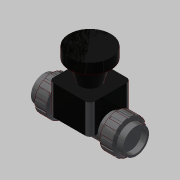
# Autodesk Inventor part: DIAPHRAGM VALVE MANUAL GLUED DN50
Saved by Autodesk Inventor 2017 (Build 210142000, 142)
## iProperties
Created: 2016-04-26
Part Number: DIAPHRAGM VALVE MANUAL GLUED DN50
Description: DKUIV
Document SubType Name: Modeling
Manufacturer: SEKISUI
Mass: 197.859 g
Surface Area: 285.44 cm^2
Volume: 153.379 cm^3
Density: 1.29 g/cm^3
Material: PVC
Appearance: Smooth - White(2)
Catalog Web Link: http://www.pocketbrewery.com
Title: BALL VALVE PVC-U TRD DN15
Autodesk Inventor part; units mm, degrees
ref_plane "YZ Plane" through (0, 0, 0) normal (1, 0, 0) x (0, 1, 0)
ref_plane "XZ Plane" through (0, 0, 0) normal (0, 1, 0) x (-1, 0, 0)
ref_plane "XY Plane" through (0, 0, 0) normal (0, 0, 1) x (1, 0, 0)
sketch "Sketch_1" plane through (0, 0, 0) normal (1, 0, 0) x (0, 1, 0)
  line L0 (116.9615, 0) -> (116.9615, -32.6667)
  line L1 (116.9615, -32.6667) -> (111.0167, -49)
  line L2 (111.0167, -49) -> (77.6193, -49)
  line L3 (77.6193, -49) -> (74.7393, -41.0872)
  line L4 (74.7393, -41.0872) -> (74.7393, -32.6667)
  line L5 (-74.7393, -32.6667) -> (-74.7393, -41.0872)
  line L6 (-74.7393, -41.0872) -> (-77.6193, -49)
  line L7 (-77.6193, -49) -> (-111.0167, -49)
  line L8 (-111.0167, -49) -> (-116.9615, -32.6667)
  line L9 (-116.9615, -32.6667) -> (-116.9615, 0)
  line L10 (-116.9615, 0) -> (116.9615, 0)
  line L11 (-77.6193, -49) -> (0, -49) construction
  line L12 (0, -49) -> (0, -50.7038) construction
  line L13 (-111.7446, -49) -> (-79.6193, -49)
  line L14 (-79.6193, -49) -> (-79.6193, -47)
  line L15 (-79.6193, -47) -> (-111.7446, -47)
  line L16 (-111.7446, -47) -> (-111.7446, -49)
  line L17 (79.6193, -49) -> (111.7446, -49)
  line L18 (111.7446, -49) -> (111.7446, -47)
  line L19 (111.7446, -47) -> (79.6193, -47)
  line L20 (79.6193, -47) -> (79.6193, -49)
  line L21 (-74.7393, -32.6667) -> (74.7393, -32.6667)
  point P0 (0, 0)
  point P1 (0, 0)
  point P2 (-94.318, -49)
  point P3 (95.682, -49)
  point P4 (0, 0)
  dimension "dimE" = 98
  dimension "d22" = 49
  dimension "d23" = 16.3333
  dimension "d24" = 20
  dimension "d27" = 42.2222
  dimension "d28" = 42.2222
  dimension "d52" = 20
  dimension "d53" = 2
  dimension "d54" = 2
  dimension "d55" = 2
  dimension "dimZ" = 190
  constraints: 44 end point, 6 parallel, 5 equal length, 5 horizontal, 5 perpendicular, 4 point on line, 3 collinear, 3 midpoint, 2 coincident
  measures "dimE" diameter of L2 L10
  measures "d22" distance from line of L0.start L2
  measures "d23" vertical distance of L0.end L1.end
  measures "d24" angle of L0 L1
  measures "d27" distance between parallel lines of L9 L5
  measures "d28" distance between parallel lines of L0 L4
  measures "d52" angle of L5 L6
  measures "d53" distance of L15.end L13.start
  measures "d54" distance from line of L6.end L14
  measures "d55" distance from line of L2.end L20
  measures "dimZ" distance of point (95.682, -49) point (-94.318, -49)
revolve "Revolution1" add sketch "Sketch_1" angle 360 about axis through (0, -116.9615, 0) along (0, 1, 0) contours L0 L1 L19 L20 L2 L3 L4 L21 L5 L6 L7 L14 L15 L8 L9 L10 | L1 L2 L20 L19 | L15 L14 L7 L8 | L8 L13 L16
sketch "Sketch11" plane through (0, 0, 0) normal (0, 0, 1) x (1, 0, 0)
  line L0 (-59.7393, 59.7393) -> (59.7393, 59.7393)
  line L1 (59.7393, 59.7393) -> (59.7393, -59.7393)
  line L2 (59.7393, -59.7393) -> (-59.7393, -59.7393)
  line L3 (-59.7393, -59.7393) -> (-59.7393, 59.7393)
  line L4 (59.7393, -59.7393) -> (-59.7393, 59.7393)
  line L5 (41.0872, 74.7393) -> (-41.0872, 74.7393) projected
  point P0 (0, 0)
  point P1 (0, 0)
  point P2 (0, 0)
  dimension "d67" = 15
  constraints: 10 end point, 2 coincident, 2 parallel, 2 perpendicular, 1 horizontal, 1 midpoint
  measures "d67" distance between parallel lines of L0 L5
extrude "Extrusion6" add sketch "Sketch11" along normal blind 86
sketch "Sketch_2" plane through (0, 0, 0) normal (1, 0, 0) x (0, 1, 0)
  line L0 (0, 0) -> (0, 172)
  line L1 (0, 172) -> (30, 172)
  line L2 (30, 172) -> (30, 0)
  line L3 (30, 0) -> (0, 0)
  line L4 (0, 0) -> (0, 172)
  line L5 (0, 172) -> (60, 172)
  line L6 (60, 172) -> (60, 142)
  line L7 (60, 142) -> (0, 142)
  line L8 (0, 142) -> (0, 172)
  line L9 (30, 86) -> (30, 142)
  line L10 (30, 142) -> (60, 142)
  line L11 (60, 142) -> (52.2105, 139.9128)
  arc A0 (52.2105, 139.9128) -> (41.6039, 129.3062) centre (56.0927, 125.4239) ccw
  line L12 (41.6039, 129.3062) -> (30, 86)
  dimension "dimB" = 172
  dimension "dimH1" = 120
  dimension "d60" = 30
  dimension "d61" = 30
  dimension "d65" = 15
  dimension "d66" = 15
  dimension "d68" = 15
  constraints: 26 end point, 4 perpendicular, 3 midpoint, 2 parallel, 2 point on circle, 2 tangent, 1 centre point, 1 coincident, 1 horizontal, 1 vertical
  measures "dimB" distance of L0.start L0.end
  measures "dimH1" diameter of L6 L8
  measures "d60" distance of L5.end L6.end
  measures "d61" distance between parallel lines of L0 L2
  measures "d65" angle of L9 L12
  measures "d66" radius of A0
  measures "d68" angle of L7 L11
revolve "Revolution2" add sketch "Sketch_2" angle 360 about axis through (0, 0, 0) along (0, 0, -1)
fillet "Fillet1" radius 13.4 4 edges at (-59.7393, 59.7393, 43) (-59.7393, -59.7393, 43) (59.7393, -59.7393, 43) (59.7393, 59.7393, 43)
sketch "Sketch_7" plane through (0, 0, 0) normal (1, 0, 0) x (0, 1, 0)
  line L0 (-133, 37.5) -> (133, 37.5)
  line L1 (43.6087, 0) -> (-43.6087, 0)
  line L2 (-133, 37.5) -> (-133, 31.5)
  line L3 (-133, 31.5) -> (133, 31.5)
  line L4 (133, 31.5) -> (133, 37.5)
  line L5 (0, -4.2419) -> (0, 47.4898)
  point P0 (0, 0)
  point P1 (0, 0)
  point P2 (0, 31.5)
  dimension "dimH" = 266
  dimension "dimD" = 63
  dimension "dimD2" = 75
  constraints: 12 end point, 3 perpendicular, 2 midpoint, 2 point on line, 1 coincident, 1 horizontal, 1 parallel, 1 vertical
  measures "dimH" distance of L2.end L3.end
  measures "dimD" diameter of L3 L1
  measures "dimD2" diameter of L0 L1
revolve "Revolution3" add sketch "Sketch_7" angle 360 about axis through (0, 43.6087, 0) along (0, -1, 0)
extrude "Extrusion8" cut sketch "Sketch_1" along normal mid plane 6.5333 contours L18 L17 L1 | L1 L2 L20 L19 | L15 L14 L7 L8 | L8 L13 L16
pattern_circular "Circular Pattern1" count 14 over 360 about axis through (0, 66.5, 0) along (0, -1, 0) of "Extrusion8"
equation "\"d23\" = 0.333333 * d22"
equation "\"d27\" = 0.222222 * dimZ"
equation "\"d28\" = d27"
equation "\"d61\" = 0.25 * dimH1"
equation "\"d35\" = 0.1 * dimC"
equation "\"d47\" = 0.0666667 * dimE"
equation "\"dimC\" = 134"
body "Solid1"
